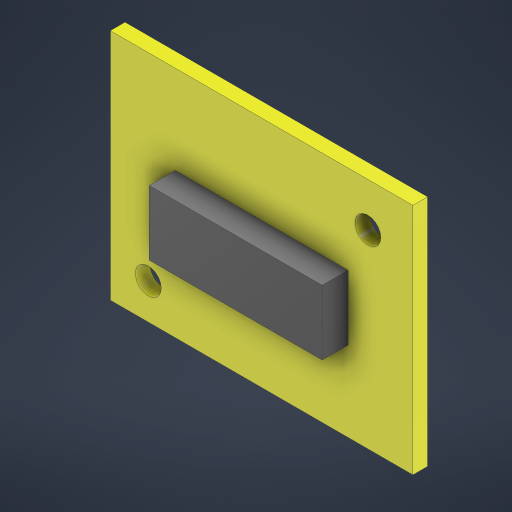
# Autodesk Inventor part: 293D
Saved by Autodesk Inventor 2024.2 (Build 282272000, 272)
## iProperties
Created: 2024-06-03
Part Number: 293D
Material: Generic
Document SubType Name: Modeling
Designer: simon
Density: 1 g/cm^3
Appearance: Default
Author: simon
Autodesk Inventor part; units mm, degrees
ref_plane "YZ Plane" through (0, 0, 0) normal (1, 0, 0) x (0, 1, 0)
ref_plane "XZ Plane" through (0, 0, 0) normal (0, 1, 0) x (-1, 0, 0)
ref_plane "XY Plane" through (0, 0, 0) normal (0, 0, 1) x (1, 0, 0)
sketch "Sketch1" plane through (0, 0, 0) normal (0, 0, 1) x (1, 0, 0)
  line L0 (0, 0) -> (35, 0)
  line L1 (35, 0) -> (35, 27)
  line L2 (35, 27) -> (0, 27)
  line L3 (0, 27) -> (0, 0)
  circle A0 centre (4.4, 4.14) radius 1.5
  circle A1 centre (29.8, 21.92) radius 1.5
  dimension "d0" = 35
  dimension "d1" = 27
  dimension "d2" = 3
  dimension "d3" = 3
  dimension "d4" = 25.4
  dimension "d5" = 4.4
  dimension "d6" = 5.08
  dimension "d7" = 17.78
  constraints: 8 end point, 2 centre point, 2 parallel, 1 horizontal, 1 perpendicular
  measures "d0" distance of L2.end L1.end
  measures "d1" distance of L1.end L0.end
  measures "d2" diameter of A0
  measures "d3" diameter of A1
  measures "d4" horizontal distance of A1.centre A0.centre
  measures "d5" distance from line of L3 A0.centre
  measures "d6" distance from line of A1.centre L2
  measures "d7" vertical distance of A0.centre A1.centre
extrude "Extrusion1" add sketch "Sketch1" along normal blind 1.7
sketch "Sketch2" plane through (0, 0, 1.7) normal (0, 0, 1) x (1, 0, 0)
  line L0 (7.5, 16.75) -> (27.5, 16.75)
  line L1 (27.5, 16.75) -> (27.5, 9.25)
  line L2 (27.5, 9.25) -> (7.5, 9.25)
  line L3 (7.5, 9.25) -> (7.5, 16.75)
  line L4 (0, 27) -> (0, 0) projected
  line L5 (35, 0) -> (35, 27) projected
  line L6 (35, 27) -> (0, 27) projected
  point P0 (27.5, 13)
  point P1 (17.5, 16.75)
  dimension "d10" = 7.5
  dimension "d11" = 7.5
  dimension "d12" = 7.5
  dimension "d13" = 10.25
  constraints: 8 end point, 2 midpoint, 2 parallel, 1 horizontal, 1 perpendicular
  measures "d10" distance between parallel lines of L4 L3
  measures "d11" distance from line of L5 point (27.5, 13)
  measures "d12" distance from line of point (17.5, 16.75) L2
  measures "d13" distance between parallel lines of L6 L0
extrude "Extrusion2" add sketch "Sketch2" along normal blind 3
body "Solid1"
